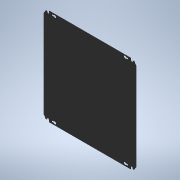
# Autodesk Inventor part: CAD_MPL_1054.000
Saved by Autodesk Inventor 2021 (Build 250183000, 183)
## iProperties
Created: 2025-08-26
Part Number: CAD_MPL_1054.000
Material: Generic
Catalog Web Link: www.cadenas.de
Description: Mounting plate AE 2.0-Mounting plate AE 2.0
Vendor: RITTAL
Document SubType Name: Modeling
Designer: psAdmin
Manufacturer: RITTAL
Mass: 783.302 g
Surface Area: 6330.76 cm^2
Volume: 783.302 cm^3
Density: 1 g/cm^3
Appearance: PSOLRGB-175-175-175
Category: PARTsolutions
Company: RITTAL
Title: CAD_MPL_1054.000
Author: Cadenas PARTsolutions
Comments: Mounting plate AE 2.0
PSOL_IDENT_0: {$CADENAS_DATA/23d-libs/rittal/schaltschranksys/ausbauteile_cad/montageplatten/ae_2_0_sep_mpl.prj},1
PSOL_IDENT_1: 88 {VTYP=3D},{NB=CAD_MPL_1054.000},{LINA=CAD_MPL_1054.000},{NN=Mounting plate AE 2.0},{DATE=28.04.20
PSOL_IDENT_2: 25 21:10:24},{GEOMDATE=11.04.2025 11:21:17},{VERSION=},{LINEID=540},{WBVAR=},{WBNUMERIC=}  {NB=CAD_M
PSOL_IDENT_3: PL_1054.000},{LINA=CAD_MPL_1054.000},{KT=DUMMY},{BEST=CAD_MPL_1054.000},{BEST2=1054.000},{B=600},{H=
PSOL_IDENT_4: 600},{T=MIN},{B1=550},{H1=575},{VERS=3},{DETAIL=1},{BEZ1=Neues Kompaktgehäuse},{BEZ2=Stahlblech},{BE
PSOL_IDENT_5: Z3=eintürig},{F=550},{G=575},{S=2.5},{CNSECLASS51=27-18-01-02},{CNSECLASS70=27-18-01-01},{CNSECLASS8
PSOL_IDENT_6: 0=27-18-01-01},{CNSETIM40=EC000261},{GEW=0}
NB: CAD_MPL_1054.000
NN: Mounting plate AE 2.0
NT: Mounting plate AE 2.0
NBSYN: $BEST.
LINA: CAD_MPL_1054.000
CATALOG: Rittal
BEST: CAD_MPL_1054.000
F: 550
G: 575
S: 2.5
GEW: 0
SUPPLIER: RITTAL
ARTICLENO: CAD_MPL_1054.000
BOMINFO: CAD_MPL_1054.000
CREATOR: CADENAS GmbH
Autodesk Inventor part; units mm, degrees
sketch "Sketch_11" plane through (0, 0, 0) normal (0, 0, 1) x (1, 0, 0)
  line L0 (-275, 538.5) -> (-275, 11.5)
  line L1 (-275, 11.5) -> (-274.0774, 11.5)
  arc A0 (-273.2113, 11) -> (-274.0774, 11.5) centre (-274.0774, 10.5) ccw
  line L2 (-273.2113, 11) -> (-264.2624, -4.5)
  arc A1 (-264.2624, -4.5) -> (-263.3964, -5) centre (-263.3964, -4) ccw
  line L3 (-263.3964, -5) -> (-256.5, -5)
  arc A2 (-256.5, -5) -> (-255.5, -4) centre (-256.5, -4) ccw
  line L4 (-255.5, -4) -> (-255.5, 0)
  arc A3 (-244.5, 0) -> (-255.5, 0) centre (-250, 0) ccw
  line L5 (-244.5, 0) -> (-244.5, -11)
  line L6 (-244.5, -11) -> (-243, -12.5)
  line L7 (-243, -12.5) -> (243, -12.5)
  line L8 (243, -12.5) -> (244.5, -11)
  line L9 (244.5, -11) -> (244.5, 0)
  arc A4 (255.5, 0) -> (244.5, 0) centre (250, 0) ccw
  line L10 (255.5, 0) -> (255.5, -4)
  arc A5 (255.5, -4) -> (256.5, -5) centre (256.5, -4) ccw
  line L11 (256.5, -5) -> (263.3964, -5)
  arc A6 (263.3964, -5) -> (264.2624, -4.5) centre (263.3964, -4) ccw
  line L12 (264.2624, -4.5) -> (273.2113, 11)
  arc A7 (274.0774, 11.5) -> (273.2113, 11) centre (274.0774, 10.5) ccw
  line L13 (274.0774, 11.5) -> (275, 11.5)
  line L14 (275, 11.5) -> (275, 538.5)
  line L15 (275, 538.5) -> (274.0774, 538.5)
  arc A8 (273.2113, 539) -> (274.0774, 538.5) centre (274.0774, 539.5) ccw
  line L16 (273.2113, 539) -> (264.2624, 554.5)
  arc A9 (264.2624, 554.5) -> (263.3964, 555) centre (263.3964, 554) ccw
  line L17 (263.3964, 555) -> (256.5, 555)
  arc A10 (256.5, 555) -> (255.5, 554) centre (256.5, 554) ccw
  line L18 (255.5, 554) -> (255.5, 550)
  arc A11 (244.5, 550) -> (255.5, 550) centre (250, 550) ccw
  line L19 (244.5, 550) -> (244.5, 561)
  line L20 (244.5, 561) -> (243, 562.5)
  line L21 (243, 562.5) -> (-243, 562.5)
  line L22 (-243, 562.5) -> (-244.5, 561)
  line L23 (-244.5, 561) -> (-244.5, 550)
  arc A12 (-255.5, 550) -> (-244.5, 550) centre (-250, 550) ccw
  line L24 (-255.5, 550) -> (-255.5, 554)
  arc A13 (-255.5, 554) -> (-256.5, 555) centre (-256.5, 554) ccw
  line L25 (-256.5, 555) -> (-263.3964, 555)
  arc A14 (-263.3964, 555) -> (-264.2624, 554.5) centre (-263.3964, 554) ccw
  line L26 (-264.2624, 554.5) -> (-273.2113, 539)
  arc A15 (-274.0774, 538.5) -> (-273.2113, 539) centre (-274.0774, 539.5) ccw
  line L27 (-274.0774, 538.5) -> (-275, 538.5)
  arc A16 (216.5296, 4.6222) -> (216.5296, -4.6222) centre (210, 0) ccw
  arc A17 (217.3457, -4.2) -> (216.5296, -4.6222) centre (217.3457, -5.2) ccw
  line L28 (217.3457, -4.2) -> (228, -4.2)
  arc A18 (228, -4.2) -> (229, -3.2) centre (228, -3.2) ccw
  line L29 (229, -3.2) -> (229, 3.2)
  arc A19 (229, 3.2) -> (228, 4.2) centre (228, 3.2) ccw
  line L30 (228, 4.2) -> (217.3457, 4.2)
  arc A20 (216.5296, 4.6222) -> (217.3457, 4.2) centre (217.3457, 5.2) ccw
  arc A21 (216.5296, 554.6222) -> (216.5296, 545.3778) centre (210, 550) ccw
  arc A22 (217.3457, 545.8) -> (216.5296, 545.3778) centre (217.3457, 544.8) ccw
  line L31 (217.3457, 545.8) -> (228, 545.8)
  arc A23 (228, 545.8) -> (229, 546.8) centre (228, 546.8) ccw
  line L32 (229, 546.8) -> (229, 553.2)
  arc A24 (229, 553.2) -> (228, 554.2) centre (228, 553.2) ccw
  line L33 (228, 554.2) -> (217.3457, 554.2)
  arc A25 (216.5296, 554.6222) -> (217.3457, 554.2) centre (217.3457, 555.2) ccw
  line L34 (-229, 3.2) -> (-229, -3.2)
  arc A26 (-229, -3.2) -> (-228, -4.2) centre (-228, -3.2) ccw
  line L35 (-228, -4.2) -> (-217.3457, -4.2)
  arc A27 (-216.5296, -4.6222) -> (-217.3457, -4.2) centre (-217.3457, -5.2) ccw
  arc A28 (-216.5296, -4.6222) -> (-216.5296, 4.6222) centre (-210, 0) ccw
  arc A29 (-217.3457, 4.2) -> (-216.5296, 4.6222) centre (-217.3457, 5.2) ccw
  line L36 (-217.3457, 4.2) -> (-228, 4.2)
  arc A30 (-228, 4.2) -> (-229, 3.2) centre (-228, 3.2) ccw
  arc A31 (-229, 546.8) -> (-228, 545.8) centre (-228, 546.8) ccw
  line L37 (-228, 545.8) -> (-217.3457, 545.8)
  arc A32 (-216.5296, 545.3778) -> (-217.3457, 545.8) centre (-217.3457, 544.8) ccw
  arc A33 (-216.5296, 545.3778) -> (-216.5296, 554.6222) centre (-210, 550) ccw
  arc A34 (-217.3457, 554.2) -> (-216.5296, 554.6222) centre (-217.3457, 555.2) ccw
  line L38 (-217.3457, 554.2) -> (-228, 554.2)
  arc A35 (-228, 554.2) -> (-229, 553.2) centre (-228, 553.2) ccw
  line L39 (-229, 553.2) -> (-229, 546.8)
  constraints: 80 end point, 72 point on circle, 36 centre point
extrude "Extrusion1" add sketch "Sketch_11" against normal blind 2.5
ref_plane "MP_XY" through (0, 0, 0) normal (0, 0, 1) x (1, 0, 0)
ref_plane "MP_YZ" through (0, 0, 0) normal (1, 0, 0) x (0, 1, 0)
ref_plane "MP_ZX" through (0, 0, 0) normal (0, 1, 0) x (0, 0, 1)
ref_plane "to_EB_XY" through (224.8, 0, -2.5) normal (0, 0, 1) x (1, 0, 0)
ref_plane "to_EB_YZ" through (224.8, 0, -2.5) normal (1, 0, 0) x (0, 1, 0)
ref_plane "to_EB_ZX" through (224.8, 0, -2.5) normal (0, 1, 0) x (0, 0, 1)
body "Solid1"
